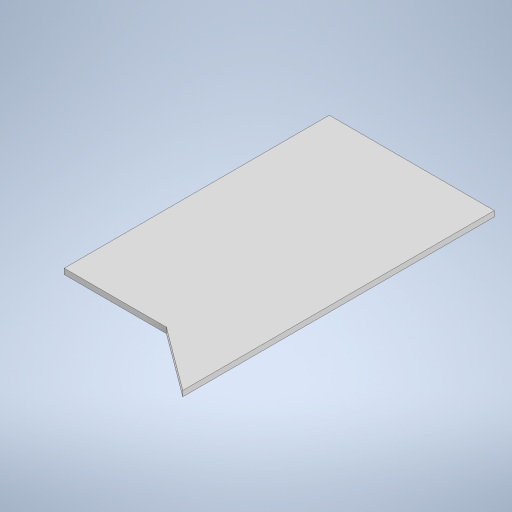
# Autodesk Inventor part: tapa4
Saved by Autodesk Inventor 2024 (Build 280153000, 153)
## iProperties
Created: 2024-05-27
Part Number: tapa4
Material: Generic
Document SubType Name: Modeling
Designer: samue
Density: 1 g/cm^3
Appearance: Default
Author: samue
## iProperties of the stored document tapa4_3DPrint.ipt
Created: 2024-05-27
Part Number: tapa4_3DPrint
Material: Generic
Document SubType Name: Modeling
Designer: samue
Density: 1 g/cm^3
Appearance: Default
Author: samue
Autodesk Inventor part; units mm, degrees
ref_plane "YZ Plane" through (0, 0, 0) normal (1, 0, 0) x (0, 1, 0)
ref_plane "XZ Plane" through (0, 0, 0) normal (0, 1, 0) x (-1, 0, 0)
ref_plane "XY Plane" through (0, 0, 0) normal (0, 0, 1) x (1, 0, 0)
sketch "Sketch1" plane through (0, 0, 0) normal (0, 1, 0) x (-1, 0, 0)
  line L0 (0, 13.9753) -> (0, -99.2247)
  line L1 (0, -99.2247) -> (60, -99.2247)
  line L2 (0, 13.9753) -> (23, -3.0438)
  line L3 (23, -3.0438) -> (60, -3.0438)
  line L4 (60, -3.0438) -> (60, -99.2247)
  point P0 (0, 0)
  dimension "d0" = 113.2
  dimension "d2" = 60
  dimension "d5" = 53.5
  dimension "d6" = 37
  constraints: 10 end point, 2 perpendicular, 1 horizontal, 1 vertical
  measures "d0" distance of L0.start L0.end
  measures "d2" distance of L0.end L1.end
  measures "d5" angle of L0 L2
  measures "d6" distance of L2.end L3.end
extrude "Extrusion1" add sketch "Sketch1" along normal blind 2
sketch "Sketch2" plane through (-60, 0, -3.0438) normal (0, 0, 1) x (1, 0, 0)
  line L0 (0, 0) -> (0, 2) projected
  line L1 (60, 0) -> (0, 0) projected
  line L2 (0, 2) -> (37, 2)
  line L3 (37, 2) -> (37, 0)
  line L4 (37, 0) -> (0, 0)
  line L5 (0, 0) -> (0, 2)
  line L6 (37, 0) -> (37, 2) projected
  point P0 (37, 1)
  constraints: 8 end point, 2 midpoint, 2 parallel, 1 horizontal, 1 perpendicular, 1 point on line
extrude "Extrusion2" add sketch "Sketch2" along normal blind 0.1
body "Solid1"
